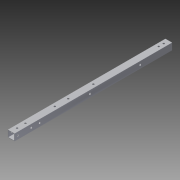
# Autodesk Inventor part: Rebuild Edge Mount 4
Saved by Autodesk Inventor 2014 SP1 (Build 180222100, 222)
## iProperties
Created: 2013-01-31
Part Number: Rebuild Edge Mount 4
Material: Aluminum 6061
Document SubType Name: Modeling
Designer: actoennies
Mass: 240.922 g
Surface Area: 1131.09 cm^2
Volume: 88.901 cm^3
Density: 2.71 g/cm^3
Appearance: Aluminum - Flat
Author: actoennies
Autodesk Inventor part; units mm, degrees
ref_plane "YZ Plane" through (0, 0, 0) normal (1, 0, 0) x (0, 1, 0)
ref_plane "XZ Plane" through (0, 0, 0) normal (0, 1, 0) x (-1, 0, 0)
ref_plane "XY Plane" through (0, 0, 0) normal (0, 0, 1) x (1, 0, 0)
sketch "Sketch1" plane through (0, 0, 0) normal (0, 0, 1) x (1, 0, 0)
  line L0 (0, 0) -> (25.4, 0)
  line L1 (25.4, 0) -> (25.4, 25.4)
  line L2 (25.4, 25.4) -> (0, 25.4)
  line L3 (0, 25.4) -> (0, 0)
  line L4 (1.5875, 23.8125) -> (23.8125, 23.8125)
  line L5 (23.8125, 23.8125) -> (23.8125, 1.5875)
  line L6 (23.8125, 1.5875) -> (1.5875, 1.5875)
  line L7 (1.5875, 1.5875) -> (1.5875, 23.8125)
  dimension "d0" = 25.4
  dimension "d2" = 25.4
  dimension "d3" = 1.5875
  constraints: 16 end point, 4 parallel, 2 perpendicular, 1 horizontal, 3 other
  measures "d0" distance of L1.end L2.end
  measures "d2" distance of L0.end L1.end
  measures "d3" distance between parallel lines of L2 L4
extrude "Extrusion1" add sketch "Sketch1" along normal blind 596.9
sketch "Sketch3" plane through (0, 0, 0) normal (0, -1, 0) x (1, 0, 0)
  circle A0 centre (12.7, 574.675) radius 3.3782 projected
  circle A1 centre (12.7, 542.925) radius 3.3782 projected
  circle A2 centre (12.7, 19.05) radius 3.302 projected
  circle A3 centre (12.7, 38.1) radius 3.302 projected
  arc A4 (3.175, 50.8) -> (0, 47.625) centre (3.175, 47.625) ccw projected
  line L0 (3.175, 50.8) -> (22.225, 50.8) projected
  arc A5 (25.4, 47.625) -> (22.225, 50.8) centre (22.225, 47.625) ccw projected
  line L1 (25.4, 47.625) -> (25.4, 4.445) projected
  line L2 (25.4, 4.445) -> (0, 4.445) projected
  line L3 (0, 47.625) -> (0, 4.445) projected
  circle A6 centre (12.7, 431.8) radius 3.3782 projected
  circle A7 centre (12.7, 381) radius 3.3782 projected
  circle A8 centre (12.7, 285.75) radius 3.3782 projected
extrude "Extrusion3" cut sketch "Sketch3" against normal blind 25.4 contours A0 | A1 | A2 | A3 | A6 | A7 | A8
sketch "Sketch4" plane through (0, 0, 0) normal (-1, 0, 0) x (0, 0, 1)
  circle A0 centre (533.4, 12.7) radius 3.3782 projected
  circle A1 centre (584.2, 12.7) radius 3.3782 projected
  line L0 (0, 25.4) -> (0, 0) projected
  line L1 (596.9, 25.4) -> (596.9, 0) projected
  line L2 (596.9, 12.7) -> (0, 12.7) construction
  circle A2 centre (501.65, 12.7) radius 3.3782
  circle A3 centre (311.15, 12.7) radius 3.3782
  circle A4 centre (120.65, 12.7) radius 3.3782
  dimension "d12" = 31.75
  dimension "d15" = 190.5
  constraints: 3 centre point, 2 end point, 2 midpoint, 1 equal radius, 1 horizontal, 1 point on line, 4 other
  measures "d12" distance of A0.centre A2.centre
  measures "d15" distance of A2.centre A3.centre
extrude "Extrusion4" cut sketch "Sketch4" against normal blind 25.4
body "Solid1"
